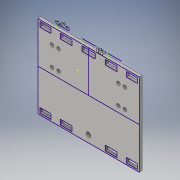
# Autodesk Inventor part: mcdave_frame
Saved by Autodesk Inventor 2016 (Build 200138000, 138)
## iProperties
Created: 2017-11-27
Part Number: mcdave_frame
Material: Generic
Document SubType Name: Modeling
Designer: student
Density: 1 g/cm^3
Appearance: Default
Author: student
Autodesk Inventor part; units mm, degrees
ref_plane "YZ Plane" through (0, 0, 0) normal (1, 0, 0) x (0, 1, 0)
ref_plane "XZ Plane" through (0, 0, 0) normal (0, 1, 0) x (-1, 0, 0)
ref_plane "XY Plane" through (0, 0, 0) normal (0, 0, 1) x (1, 0, 0)
sketch "Sketch1" plane through (0, 0, 0) normal (0, 0, 1) x (1, 0, 0)
  line L0 (-32.1176, 19.9326) -> (49.1624, 19.9326)
  line L1 (49.1624, 19.9326) -> (49.1624, -46.1074)
  line L2 (49.1624, -46.1074) -> (-32.1176, -46.1074)
  line L3 (-32.1176, -46.1074) -> (-32.1176, 19.9326)
  circle A0 centre (8.5224, -40.4127) radius 1.905
  circle A1 centre (32.4792, -8.3485) radius 1.4351
  circle A2 centre (32.4792, -8.3485) radius 1.4351
  circle A3 centre (32.4734, 7.2247) radius 1.4292
  circle A4 centre (37.7095, 7.2188) radius 1.4355
  circle A5 centre (37.7095, 7.2188) radius 1.4355
  circle A6 centre (37.7197, -8.3485) radius 1.4351
  circle A7 centre (32.4794, 7.2247) radius 1.4351
  circle A8 centre (-15.4344, -8.3485) radius 1.4351
  circle A9 centre (-15.4344, -8.3485) radius 1.4351
  circle A10 centre (-15.4286, 7.2247) radius 1.4292
  circle A11 centre (-20.6647, 7.2188) radius 1.4355
  circle A12 centre (-20.6647, 7.2188) radius 1.4355
  circle A13 centre (-20.6749, -8.3485) radius 1.4351
  circle A14 centre (-15.4345, 7.2247) radius 1.4351
  point P0 (0, 0)
  dimension "d0" = 81.28
  dimension "d1" = 66.04
  dimension "d2" = 3.81
  constraints: 15 centre point, 8 end point, 4 coincident, 2 parallel, 1 horizontal, 1 perpendicular, 1 tangent
  measures "d0" distance of L0.start L0.end
  measures "d1" distance of L0.end L1.end
  measures "d2" diameter of A0
extrude "Extrusion1" add sketch "Sketch1" along normal blind 2.286 contours L0 L1 L2 L3
sketch "Sketch2" plane through (0, 0, 2.286) normal (0, 0, 1) x (1, 0, 0)
  line L0 (49.1624, -46.1074) -> (49.1624, 19.9326) projected
  line L1 (49.1624, -13.0874) -> (-32.1176, -13.0874)
  line L2 (-32.1176, 19.9326) -> (-32.1176, -46.1074) projected
  line L3 (-32.1176, -46.1074) -> (49.1624, -46.1074) projected
  line L4 (49.1624, 19.9326) -> (-32.1176, 19.9326) projected
  line L5 (47.5774, -44.8414) -> (47.5774, -40.9552)
  line L6 (47.5774, -44.8414) -> (38.8489, -44.8414)
  line L7 (38.8489, -44.8414) -> (38.8489, -40.9552)
  line L8 (38.8489, -40.9552) -> (47.5774, -40.9552)
  line L9 (-30.5326, -44.8414) -> (-30.5326, -40.9552)
  line L10 (-30.5326, -44.8414) -> (-21.804, -44.8414)
  line L11 (-21.804, -44.8414) -> (-21.804, -40.9552)
  line L12 (-21.804, -40.9552) -> (-30.5326, -40.9552)
  line L13 (31.2541, -44.8414) -> (31.2541, -40.9552)
  line L14 (31.2541, -40.9552) -> (21.8023, -40.9552)
  line L15 (21.8023, -40.9552) -> (21.8023, -44.8414)
  line L16 (21.8023, -44.8414) -> (31.2541, -44.8414)
  line L17 (-32.1176, 19.9326) -> (49.1624, 19.9326)
  line L18 (47.5774, 18.6666) -> (47.5774, 14.7804)
  line L19 (47.5774, 18.6666) -> (38.8489, 18.6666)
  line L20 (38.8489, 18.6666) -> (38.8489, 14.7804)
  line L21 (38.8489, 14.7804) -> (47.5774, 14.7804)
  line L22 (-21.804, 18.6666) -> (-21.804, 14.7804)
  line L23 (-30.5326, 18.6666) -> (-21.804, 18.6666)
  line L24 (-21.804, 14.7804) -> (-30.5326, 14.7804)
  line L25 (-30.5326, 18.6666) -> (-30.5326, 14.7804)
  line L26 (31.2541, 18.6666) -> (31.2541, 14.7804)
  line L27 (31.2541, 14.7804) -> (21.8023, 14.7804)
  line L28 (21.8023, 14.7804) -> (21.8023, 18.6666)
  line L29 (21.8023, 18.6666) -> (31.2541, 18.6666)
  line L30 (-14.2093, -44.8414) -> (-14.2093, -40.9552)
  line L31 (-14.2093, -40.9552) -> (-4.7575, -40.9552)
  line L32 (-4.7575, -40.9552) -> (-4.7575, -44.8414)
  line L33 (-4.7575, -44.8414) -> (-14.2093, -44.8414)
  line L34 (-4.7575, 14.7804) -> (-4.7575, 18.6666)
  line L35 (-14.2093, 14.7804) -> (-4.7575, 14.7804)
  line L36 (-4.7575, 18.6666) -> (-14.2093, 18.6666)
  line L37 (-14.2093, 18.6666) -> (-14.2093, 14.7804)
  line L38 (13.8264, 18.6666) -> (13.8264, 14.7804)
  line L39 (3.2185, 18.6666) -> (3.2185, 14.7804)
  line L40 (13.8264, 14.7804) -> (3.2185, 14.7804)
  line L41 (13.8264, 18.6666) -> (3.2185, 18.6666)
  point P0 (0, 0)
  dimension "d15" = 3.8862
  constraints: 76 end point, 16 symmetric about line, 6 perpendicular, 3 vertical, 2 midpoint, 1 horizontal, 1 parallel
  measures "d15" distance of L5.start L5.end
extrude "Extrusion2" cut sketch "Sketch2" against normal through all contours L6 L7 L8 L5 | L9 L12 L11 L10 | L16 L15 L14 L13 | L18 L21 L20 L19 | L22 L24 L25 L23 | L26 L27 L28 L29 | L30 L31 L32 L33 | L35 L37 L36 L34 | L38 L40 L39 L41
sketch "Sketch3" plane through (0, 0, 2.286) normal (0, 0, 1) x (1, 0, 0)
  line L0 (49.1624, -46.1074) -> (-32.1176, -46.1074) projected
  line L1 (-32.1176, 19.9326) -> (49.1624, 19.9326) projected
  line L2 (49.1624, 19.9326) -> (49.1624, -46.1074) projected
  line L3 (49.1624, -13.0874) -> (-32.1176, -13.0874)
  line L4 (-32.1176, -46.1074) -> (-32.1176, 19.9326) projected
  point P0 (0, 0)
  constraints: 2 end point, 2 midpoint
sketch "Sketch4" plane through (0, 0, 2.286) normal (0, 0, 1) x (1, 0, 0)
  line L0 (49.1624, -46.1074) -> (-32.1176, -46.1074) projected
  line L1 (49.1624, 19.9326) -> (49.1624, -46.1074) projected
  line L2 (49.1624, -46.1074) -> (49.1624, 19.9326)
  line L3 (-32.1176, 19.9326) -> (49.1624, 19.9326) projected
  line L4 (49.1624, 19.9326) -> (-32.1176, 19.9326)
  line L5 (-32.1176, -46.1074) -> (-32.1176, 19.9326) projected
  line L6 (-32.1176, 19.9326) -> (-32.1176, -46.1074)
  line L7 (-32.1176, -46.1074) -> (49.1624, -46.1074)
  line L8 (47.5774, -44.8414) -> (38.8489, -44.8414) projected
  line L9 (47.5774, -44.8414) -> (38.8489, -44.8414)
  line L10 (38.8489, -40.9552) -> (38.8489, -44.8414) projected
  line L11 (38.8489, -44.8414) -> (38.8489, -40.9552)
  line L12 (38.8489, -40.9552) -> (47.5774, -40.9552) projected
  line L13 (38.8489, -40.9552) -> (47.5774, -40.9552)
  line L14 (47.5774, -40.9552) -> (47.5774, -44.8414) projected
  line L15 (47.5774, -40.9552) -> (47.5774, -44.8414)
  line L16 (47.5774, 14.7804) -> (38.8489, 14.7804) projected
  line L17 (47.5774, 14.7804) -> (38.8489, 14.7804)
  line L18 (38.8489, 14.7804) -> (38.8489, 18.6666) projected
  line L19 (38.8489, 14.7804) -> (38.8489, 18.6666)
  line L20 (38.8489, 18.6666) -> (47.5774, 18.6666) projected
  line L21 (38.8489, 18.6666) -> (47.5774, 18.6666)
  line L22 (47.5774, 18.6666) -> (47.5774, 14.7804) projected
  line L23 (47.5774, 18.6666) -> (47.5774, 14.7804)
  line L24 (31.2541, -44.8414) -> (21.8023, -44.8414) projected
  line L25 (31.2541, -44.8414) -> (21.8023, -44.8414)
  line L26 (21.8023, -40.9552) -> (21.8023, -44.8414) projected
  line L27 (21.8023, -44.8414) -> (21.8023, -40.9552)
  line L28 (21.8023, -40.9552) -> (31.2541, -40.9552)
  line L29 (31.2541, -40.9552) -> (31.2541, -44.8414) projected
  line L30 (31.2541, -40.9552) -> (31.2541, -44.8414)
  line L31 (-4.7575, -44.8414) -> (-14.2093, -44.8414) projected
  line L32 (-4.7575, -44.8414) -> (-14.2093, -44.8414)
  line L33 (-14.2093, -40.9552) -> (-14.2093, -44.8414) projected
  line L34 (-14.2093, -44.8414) -> (-14.2093, -40.9552)
  line L35 (-4.7575, -40.9552) -> (-14.2093, -40.9552) projected
  line L36 (-14.2093, -40.9552) -> (-4.7575, -40.9552)
  line L37 (-4.7575, -40.9552) -> (-4.7575, -44.8414) projected
  line L38 (-4.7575, -40.9552) -> (-4.7575, -44.8414)
  line L39 (-21.804, -40.9552) -> (-21.804, -44.8414) projected
  line L40 (-30.5326, -44.8414) -> (-21.804, -44.8414) projected
  line L41 (-21.804, -44.8414) -> (-30.5326, -44.8414)
  line L42 (-30.5326, -44.8414) -> (-30.5326, -40.9552)
  line L43 (-30.5326, -40.9552) -> (-21.804, -40.9552) projected
  line L44 (-30.5326, -40.9552) -> (-21.804, -40.9552)
  line L45 (-21.804, -40.9552) -> (-21.804, -44.8414)
  line L46 (31.2541, 14.7804) -> (21.8023, 14.7804) projected
  line L47 (31.2541, 14.7804) -> (21.8023, 14.7804)
  line L48 (21.8023, 14.7804) -> (21.8023, 18.6666) projected
  line L49 (21.8023, 14.7804) -> (21.8023, 18.6666)
  line L50 (21.8023, 18.6666) -> (31.2541, 18.6666) projected
  line L51 (21.8023, 18.6666) -> (31.2541, 18.6666)
  line L52 (31.2541, 18.6666) -> (31.2541, 14.7804) projected
  line L53 (31.2541, 18.6666) -> (31.2541, 14.7804)
  line L54 (3.2185, 14.7804) -> (13.8264, 14.7804) projected
  line L55 (13.8264, 14.7804) -> (3.2185, 14.7804)
  line L56 (3.2185, 18.6666) -> (3.2185, 14.7804) projected
  line L57 (3.2185, 14.7804) -> (3.2185, 18.6666)
  line L58 (3.2185, 18.6666) -> (13.8264, 18.6666) projected
  line L59 (3.2185, 18.6666) -> (13.8264, 18.6666)
  line L60 (13.8264, 14.7804) -> (13.8264, 18.6666) projected
  line L61 (13.8264, 18.6666) -> (13.8264, 14.7804)
  line L62 (-4.7575, 14.7804) -> (-14.2093, 14.7804) projected
  line L63 (-4.7575, 14.7804) -> (-14.2093, 14.7804)
  line L64 (-14.2093, 14.7804) -> (-14.2093, 18.6666) projected
  line L65 (-14.2093, 14.7804) -> (-14.2093, 18.6666)
  line L66 (-14.2093, 18.6666) -> (-4.7575, 18.6666) projected
  line L67 (-14.2093, 18.6666) -> (-4.7575, 18.6666)
  line L68 (-4.7575, 18.6666) -> (-4.7575, 14.7804)
  line L69 (-4.7575, 18.6666) -> (-4.7575, 14.7804) projected
  line L70 (-21.804, 18.6666) -> (-21.804, 14.7804) projected
  line L71 (-21.804, 14.7804) -> (-30.5326, 14.7804) projected
  line L72 (-21.804, 14.7804) -> (-30.5326, 14.7804)
  line L73 (-30.5326, 18.6666) -> (-21.804, 18.6666) projected
  line L74 (-30.5326, 14.7804) -> (-30.5326, 18.6666)
  line L75 (-30.5326, 18.6666) -> (-21.804, 18.6666)
  line L76 (-21.804, 18.6666) -> (-21.804, 14.7804)
  point P0 (0, 0)
  constraints: 80 end point, 36 collinear, 4 perpendicular
sketch "Sketch5" plane through (0, 0, 2.286) normal (0, 0, 1) x (1, 0, 0)
  line L0 (-32.1176, 19.9326) -> (49.1624, 19.9326) projected
  line L1 (8.5224, 19.9326) -> (8.5224, -12.873)
  line L2 (34.6629, 19.9326) -> (34.6629, 23.8188)
  line L3 (-17.618, 19.9326) -> (-17.618, 23.8188)
  line L4 (-0.161, 19.9326) -> (-17.618, 19.9326)
  line L5 (17.2058, 19.9326) -> (34.6629, 19.9326)
  line L6 (34.6629, 23.8188) -> (24.0248, 23.8188)
  line L7 (24.0248, 23.8188) -> (24.0248, 19.9326)
  line L8 (34.6629, 19.9326) -> (24.0248, 19.9326)
  line L9 (-17.618, 23.8188) -> (-6.9754, 23.8188)
  line L10 (-17.618, 19.9326) -> (-8.8895, 19.9326)
  line L11 (-6.9754, 19.9326) -> (-6.9754, 23.8188)
  line L12 (13.8264, 19.9326) -> (13.8264, 23.8188)
  line L13 (3.2185, 19.9326) -> (3.2185, 23.8188)
  line L14 (13.8264, 23.8188) -> (3.2185, 23.8188)
  point P0 (0, 0)
  dimension "d23" = 10.6426
  dimension "d24" = 3.8862
  dimension "d25" = 3.8862
  constraints: 28 end point, 5 point on line, 5 symmetric about line, 4 perpendicular, 3 collinear, 3 horizontal, 2 midpoint, 2 vertical
  measures "d23" distance of L3.end L9.end
  measures "d24" distance of L6.end L7.end
  measures "d25" distance of L12.start L12.end
body "Solid1"
